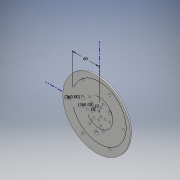
# Autodesk Inventor part: bearing-base-lower-case
Saved by Autodesk Inventor 2018 (Build 220112000, 112)
## iProperties
Created: 2025-02-23
Part Number: bearing-base-lower-case
Material: Generic
Document SubType Name: Modeling
Designer: neo
Density: 1 g/cm^3
Appearance: Default
Author: neo
Autodesk Inventor part; units mm, degrees
ref_plane "YZ Plane" through (0, 0, 0) normal (1, 0, 0) x (0, 1, 0)
ref_plane "XZ Plane" through (0, 0, 0) normal (0, 1, 0) x (-1, 0, 0)
ref_plane "XY Plane" through (0, 0, 0) normal (0, 0, 1) x (1, 0, 0)
sketch "Sketch1" plane through (0, 0, 0) normal (0, 0, 1) x (1, 0, 0)
  line L0 (18.3832, 17.5749) -> (18.3832, -20.5689)
  line L1 (68.3832, 14.8802) -> (68.3832, 4.8802) construction
  line L2 (-31.6168, 4.8802) -> (-31.6168, 14.8802) construction
  line L3 (-31.6168, 14.8802) -> (-21.6168, 14.8802) construction
  line L4 (-21.6168, 14.8802) -> (-21.6168, 4.8802) construction
  line L5 (-21.6168, 4.8802) -> (-31.6168, 4.8802) construction
  line L6 (-31.6168, 4.8802) -> (-31.6168, 14.8802) construction
  line L7 (68.3832, 14.8802) -> (-31.6168, 14.8802) construction
  line L8 (68.3832, 4.8802) -> (68.3832, 14.8802) construction
  line L9 (68.3832, 14.8802) -> (58.3832, 14.8802) construction
  line L10 (58.3832, 14.8802) -> (58.3832, 4.8802) construction
  line L11 (58.3832, 4.8802) -> (68.3832, 4.8802) construction
  line L12 (68.3832, 4.8802) -> (68.3832, 14.8802) construction
  line L13 (55.3832, 7.8802) -> (58.3832, 7.8802)
  line L14 (58.3832, 7.8802) -> (58.3832, 4.8802)
  line L15 (18.3832, 4.8802) -> (18.3832, 7.8802)
  line L16 (58.3832, 4.8802) -> (61.3832, 4.8802)
  line L17 (61.3832, 4.8802) -> (61.3832, -5.1198)
  line L18 (18.3832, -2.1198) -> (18.3832, 4.8802)
  line L19 (93.3832, -5.1198) -> (93.3832, -8.1198)
  line L20 (93.3832, -8.1198) -> (18.3832, -8.1198)
  line L21 (18.3832, -8.1198) -> (18.3832, -2.1198)
  line L22 (55.3832, 7.8802) -> (55.3832, -2.1198)
  line L23 (-31.6168, 4.8802) -> (18.3832, 4.8802) construction
  line L24 (58.3832, 4.8802) -> (68.3832, 4.8802) construction
  line L25 (18.3832, -2.1198) -> (55.3832, -2.1198)
  line L26 (61.3832, -5.1198) -> (93.3832, -5.1198)
  line L27 (58.3832, 14.8802) -> (58.3832, 4.8802) construction
  point P0 (0, 0)
  dimension "d1" = 100
  dimension "d2" = 10
  dimension "d3" = 150
  dimension "d7" = 3
  dimension "d8" = 3
  dimension "d9" = 10
  dimension "d10" = 43
  dimension "d11" = 80
  dimension "d12" = 3
  dimension "d13" = 10
  dimension "d14" = 6
  constraints: 56 end point, 8 parallel, 7 symmetric about line, 5 horizontal, 5 perpendicular, 1 point on line, 1 vertical, 1 other
  measures "d1" distance of L2.end L1.start
  measures "d2" distance between parallel lines of L2 L4
  measures "d3" diameter of L19 L0
  measures "d7" distance between parallel lines of L14 L22
  measures "d8" distance between parallel lines of L20 L26
  measures "d9" distance between parallel lines of L26 L16
  measures "d10" distance between parallel lines of L18 L17
  measures "d11" diameter of L14 L0
  measures "d12" distance between parallel lines of L16 L13
  measures "d13" distance between parallel lines of L23 L7
  measures "d14" distance between parallel lines of L20 L25
revolve "Revolution1" add sketch "Sketch1" angle 360 about axis through (18.3832, 17.5749, 0) along (0, -1, 0)
sketch "Sketch2" plane through (18.3832, -2.1198, 0) normal (0, 1, 0) x (1, 0, 0)
  circle A0 centre (0, 0) radius 37 projected
  line L0 (0, 0) -> (0, -138.0675)
  line L1 (0, 0) -> (-120, 0)
  circle A1 centre (-10, 0) radius 2
  circle A2 centre (-20, 0) radius 2
  circle A3 centre (-30, 0) radius 2
  circle A4 centre (-15, -25.9808) radius 2
  circle A5 centre (-10, -17.3205) radius 2
  circle A6 centre (-5, -8.6603) radius 2
  circle A7 centre (15, -25.9808) radius 2
  circle A8 centre (10, -17.3205) radius 2
  circle A9 centre (5, -8.6603) radius 2
  circle A10 centre (30, 0) radius 2
  circle A11 centre (20, 0) radius 2
  circle A12 centre (10, 0) radius 2
  circle A13 centre (15, 25.9808) radius 2
  circle A14 centre (10, 17.3205) radius 2
  circle A15 centre (5, 8.6603) radius 2
  circle A16 centre (-15, 25.9808) radius 2
  circle A17 centre (-10, 17.3205) radius 2
  circle A18 centre (-5, 8.6603) radius 2
  circle A19 centre (-60, 0) radius 2.5
  circle A20 centre (-30, -51.9615) radius 2.5
  circle A21 centre (30, -51.9615) radius 2.5
  circle A22 centre (60, 0) radius 2.5
  circle A23 centre (30, 51.9615) radius 2.5
  circle A24 centre (-30, 51.9615) radius 2.5
  point P0 (-18.3832, 0)
  dimension "d16" = 4
  dimension "d17" = 10
  dimension "d20" = 10
  dimension "d27" = 360
  dimension "d29" = 5
  dimension "d30" = 60
  dimension "d33" = 360
  constraints: 24 centre point, 4 end point, 2 horizontal, 1 midpoint, 1 point on line, 1 vertical, 54 other
  measures "d16" diameter of A1
  measures "d17" distance of L0.start A1.centre
  measures "d20" distance of A1.centre A2.centre
  measures "d29" diameter of A19
  measures "d30" distance of L0.start A19.centre
hole "Hole1" at (-41.6168, -2.1198, 0) at (-11.6168, -2.1198, 51.9615) at (48.3832, -2.1198, 51.9615) at (78.3832, -2.1198, 0) at (48.3832, -2.1198, -51.9615) at (-11.6168, -2.1198, -51.9615) direction (0, -1, 0) diameter 5 end through all
hole "Hole2" at (-11.6168, -2.1198, 0) at (3.3832, -2.1198, 25.9808) at (8.3832, -2.1198, 17.3205) at (13.3832, -2.1198, 8.6603) at (8.3832, -2.1198, 0) at (-1.6168, -2.1198, 0) at (8.3832, -2.1198, -17.3205) at (3.3832, -2.1198, -25.9808) at (13.3832, -2.1198, -8.6603) at (23.3832, -2.1198, -8.6603) at (28.3832, -2.1198, -17.3205) at (33.3832, -2.1198, -25.9808) at (48.3832, -2.1198, 0) at (38.3832, -2.1198, 0) at (28.3832, -2.1198, 0) at (33.3832, -2.1198, 25.9808) at (28.3832, -2.1198, 17.3205) at (23.3832, -2.1198, 8.6603) direction (0, -1, 0) diameter 4 end through all
fillet "Fillet1" radius 2 1 edges at (-24.6168, -5.1198, 0)
sketch "Sketch3" plane through (18.3832, 7.8802, 0) normal (0, 1, 0) x (1, 0, 0)
  circle A0 centre (0, 0) radius 37 projected
  circle A1 centre (0, 0) radius 40 projected
  circle A2 centre (0, 35.25) radius 1.75
  circle A3 centre (-30.5274, -17.625) radius 1.75
  circle A4 centre (30.5274, -17.625) radius 1.75
  point P0 (-18.3832, 0)
  dimension "d53" = 3.5
  dimension "d56" = 360
  constraints: 3 centre point, 1 tangent, 7 other
  measures "d53" diameter of A2
extrude "Extrusion1" cut sketch "Sketch3" against normal through all contours A2 | A3 | A4
chamfer "Chamfer2" distance 2 angle 45 3 edges at (47.1606, -8.1198, 17.625) (16.6332, -8.1198, -35.25) (-13.8942, -8.1198, 17.625)
body "Solid1"
